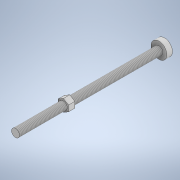
# Autodesk Inventor part: tornillo M5 largo
Saved by Autodesk Inventor 2020 (Build 240168000, 168)
## iProperties
Created: 2020-11-22
Part Number: tornillo M5 largo
Material: Generic
Document SubType Name: Modeling
Designer: michelin
Density: 1 g/cm^3
Appearance: Default
Author: michelin
Autodesk Inventor part; units mm, degrees
ref_plane "YZ Plane" through (0, 0, 0) normal (1, 0, 0) x (0, 1, 0)
ref_plane "XZ Plane" through (0, 0, 0) normal (0, 1, 0) x (-1, 0, 0)
sketch "Sketch1" plane through (0, 0, 0) normal (0, 0, 1) x (1, 0, 0)
  circle A0 centre (0, 0) radius 2.5
  circle A1 centre (0, 0) radius 5
  dimension "d12" = 5
  dimension "d18" = 10
  constraints: 2 centre point, 1 coincident
  measures "d12" diameter of A0
  measures "d18" diameter of A1
sketch "Sketch3" plane through (0, 0, 0) normal (0, 0, 1) x (1, 0, 0)
  circle A0 centre (0, 0) radius 2.5
  circle A1 centre (0, 0) radius 3.75
  dimension "d14" = 5
  dimension "d15" = 7.5
  constraints: 2 centre point, 1 coincident
  measures "d14" diameter of A0
  measures "d15" diameter of A1
extrude "Extrusion3" add sketch "Sketch3" along normal blind 90 contours A0
extrude "Extrusion4" add sketch "Sketch1" against normal blind 3.5 contours A0 | A1
thread "Thread2" size "M5x0.8" class "6g" standard "ANSI Metric M Profile" full length
ref_plane "Work Plane1" through (0, 0, 60) normal (0, 0, 1) x (1, 0, 0)
sketch "Sketch4" plane through (0, 0, 60) normal (0, 0, 1) x (1, 0, 0)
  line L0 (-3.2481, 1.8864) -> (0.0096, 3.7562)
  line L1 (0.0096, 3.7562) -> (3.2578, 1.8698)
  line L2 (3.2578, 1.8698) -> (3.2481, -1.8864)
  line L3 (3.2481, -1.8864) -> (-0.0096, -3.7562)
  line L4 (-0.0096, -3.7562) -> (-3.2578, -1.8698)
  line L5 (-3.2578, -1.8698) -> (-3.2481, 1.8864)
  point P0 (0, 0)
  point P1 (0, 0)
  constraints: 12 end point, 1 coincident, 13 other
extrude "Extrusion5" add sketch "Sketch4" against normal blind 4
body "Solid2"
